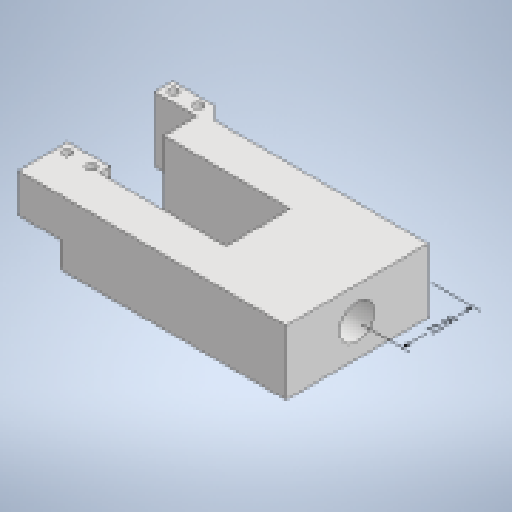
# Autodesk Inventor part: Base Catapulta
Saved by Autodesk Inventor 2024 (Build 280153000, 153)
## iProperties
Created: 2025-03-01
Part Number: Base Catapulta
Material: Genérico
Document SubType Name: Modeling
Designer: sergi
Density: 1 g/cm^3
Appearance: Valor por defecto
Author: sergi
Autodesk Inventor part; units mm, degrees
ref_plane "YZ Plane" through (0, 0, 0) normal (1, 0, 0) x (0, 1, 0)
ref_plane "XZ Plane" through (0, 0, 0) normal (0, 1, 0) x (-1, 0, 0)
ref_plane "XY Plane" through (0, 0, 0) normal (0, 0, 1) x (1, 0, 0)
sketch "Boceto1" plane through (0, 0, 0) normal (0, 1, 0) x (-1, 0, 0)
  line L0 (0, 0) -> (105, 0)
  line L1 (105, 0) -> (105, 66)
  line L2 (105, 66) -> (0, 66)
  line L3 (0, 66) -> (0, 0)
  dimension "d0" = 105
  dimension "d1" = 66
  constraints: 8 end point, 2 parallel, 1 horizontal, 1 perpendicular
  measures "d0" distance of L2.end L1.end
  measures "d1" distance of L1.end L0.end
extrude "Extrusión1" add sketch "Boceto1" along normal blind 30
sketch "Boceto2" plane through (0, 0, 66) normal (1, 0, 0) x (0, 0, -1)
  line L0 (66, 30) -> (0, 30) projected
  line L1 (0, 0) -> (66, 0) projected
  line L2 (66, 0) -> (66, 30) projected
  line L3 (0, 30) -> (66, 30) projected
  line L4 (0, 0) -> (0, 30) projected
  line L5 (66, 30) -> (0, 0)
  circle A0 centre (33, 15) radius 8.1
  dimension "d28" = 16.2
  constraints: 2 end point, 1 centre point, 1 midpoint
  measures "d28" diameter of A0
hole "Agujero1" at (0, 15, 33) direction (-1, 0, 0) diameter 16.2 depth 44
sketch "Boceto5" plane through (0, 30, 0) normal (0, 1, 0) x (1, 0, 0)
  line L0 (-105, 0) -> (-105, -66) projected
  line L1 (-105, -66) -> (0, -66) projected
  line L2 (0, -66) -> (0, 0) projected
  line L3 (0, 0) -> (-105, 0) projected
  line L4 (0, -24.9) -> (0, -41.1) projected
  line L5 (-44, -41.1) -> (-44, -24.9) projected
  line L6 (0, -41.1) -> (-44, -41.1)
  line L7 (-44, -24.9) -> (0, -24.9)
  line L8 (-46, -22.9) -> (-46, -43.1)
  line L9 (-46, -43.1) -> (2, -43.1)
  line L10 (2, -43.1) -> (2, -22.9)
  line L11 (2, -22.9) -> (-46, -22.9)
  line L12 (-46, -43.1) -> (-105, -43.1)
  line L13 (-105, 0) -> (-105, -66) projected
  line L14 (-46, -22.9) -> (-105, -22.9)
  line L15 (-105, -22.9) -> (-46, -43.1)
  line L16 (-46, -48) -> (-105, -48)
  line L17 (-105, -48) -> (-105, -18)
  line L18 (-105, -18) -> (-46, -18)
  line L19 (-46, -18) -> (-46, -48)
  line L20 (-46, -48) -> (-105, -18) construction
  line L21 (-105, -48) -> (-46, -18) construction
  point P0 (-75.5, -33)
  point P1 (-105, -18)
  dimension "d29" = 2
  dimension "d30" = 30
  constraints: 30 end point, 5 perpendicular, 4 parallel, 3 midpoint, 3 point on line, 1 horizontal, 3 other
  measures "d29" distance between parallel lines of L5 L8
  measures "d30" distance between parallel lines of L16 L18
extrude "Extrusión3" cut sketch "Boceto5" against normal through all contours L18 L19 L14 L0 | L15 L12 L0 | L14 L8 L15 | L12 L19 L16 L0
sketch "Boceto6" plane through (-46, 30, 18) normal (-1, 0, 0) x (0, 0, 1)
  circle A0 centre (20, -15) radius 1 projected
  circle A1 centre (10, -15) radius 1 projected
  point P0 (-18, -30)
hole "Agujero3" at (-46, 15, 38) at (-46, 15, 28) direction (1, 0, 0) diameter 2.2 depth 44
sketch "Boceto7" plane through (-105, 0, 66) normal (-1, 0, 0) x (0, 0, 1)
  line L0 (-18, 30) -> (-18, 0) projected
  line L1 (-18, 0) -> (0, 0) projected
  line L2 (0, 0) -> (0, 30) projected
  line L3 (-18, 30) -> (0, 30) projected
  line L4 (-68.75, 30) -> (-68.75, 32.5) projected
  line L5 (-63.6, 30) -> (-68.75, 30) projected
  line L6 (-63.6, 1.45) -> (-63.6, 30) projected
  line L7 (-23.1, 1.45) -> (-63.6, 1.45) projected
  line L8 (-23.1, 30) -> (-23.1, 1.45) projected
  line L9 (-17.95, 30) -> (-23.1, 30) projected
  line L10 (-17.95, 32.5) -> (-17.95, 30) projected
  line L11 (-23.1, 32.5) -> (-17.95, 32.5) projected
  line L12 (-23.1, 38.25) -> (-23.1, 32.5) projected
  line L13 (-33, 38.25) -> (-23.1, 38.25) projected
  line L14 (-63.6, 38.25) -> (-33, 38.25) projected
  line L15 (-63.6, 32.5) -> (-63.6, 38.25) projected
  line L16 (-68.75, 32.5) -> (-63.6, 32.5) projected
  line L17 (-23.1, 5.2) -> (-23.1, 9) projected
  line L18 (-23.1, 5.2) -> (-19.2, 5.2) projected
  line L19 (-19.2, 9) -> (-19.2, 5.2) projected
  line L20 (-23.1, 9) -> (-19.2, 9) projected
  line L21 (-23.1, 9) -> (-23.1, 12)
  line L22 (-23.1, 12) -> (0, 12)
  line L23 (-48, 0) -> (-48, 30) projected
  line L24 (-66, 30) -> (-48, 30) projected
  line L25 (-66, 0) -> (-66, 30) projected
  line L26 (-66, 0) -> (-48, 0) projected
  line L27 (-70.75, 32.5) -> (-64.75, 33.85)
  line L28 (-70.75, 32.5) -> (-70.75, 30)
  line L29 (-70.75, 32.5) -> (-70.75, 30)
  line L30 (-70.75, 30) -> (-63.6, 30)
  line L31 (-63.6, 30) -> (-63.6, 0)
  line L32 (-63.6, 0) -> (-71.95, 0)
  line L33 (-70.75, 0) -> (-70.75, 30)
  line L34 (-71.95, 31.2) -> (-62.4, 31.2)
  line L35 (-62.4, 31.2) -> (-62.4, -1.2)
  line L36 (-62.4, -1.2) -> (-71.95, -1.2)
  line L37 (-71.95, -1.2) -> (-71.95, 31.2)
  line L38 (-70.75, 0) -> (-71.95, 0)
  line L39 (-70.75, 30) -> (-71.95, 30)
  dimension "d42" = 3
  dimension "d55" = 1.2
  constraints: 30 end point, 6 point on line, 4 parallel, 4 perpendicular, 2 horizontal, 2 vertical, 5 other
  measures "d42" distance of L17.end L21.end
  measures "d55" distance between parallel lines of L33 L37
ref_plane "Plano de trabajo1" through (-124.8, 1.45, -2.75) normal (-1, 0, 0) x (0, 0, 1)
extrude "Extrusión4" add sketch "Boceto7" along normal up to surface (19.8 mm away) contours L3 L2 L22 L0 | L0 L22 L8 L9 | L31 L26 L25 L5 L6 | L25 L32 L33 L30 L5 | L32 L37 L39 L33
chamfer "Chaflán1" distance 5.95 angle 45 1 edges at (-105, 15, 0)
sketch "Boceto8" plane through (0, 30, 0) normal (0, 1, 0) x (1, 0, 0)
  circle A0 centre (-120.6, -47.5) radius 2.2 projected
  circle A1 centre (-109.2, -47.5) radius 2.2 projected
  circle A2 centre (-109.2, 2.2) radius 2.2 projected
  circle A3 centre (-120.6, 2.2) radius 2.2 projected
  point P0 (0, 0)
hole "Agujero4" at (-120.6, 30, 47.5) at (-109.2, 30, 47.5) at (-120.6, 30, -2.2) at (-109.2, 30, -2.2) direction (0, -1, 0) diameter 4.2 end through all
sketch "Boceto9" plane through (-105, 0, 66) normal (0, 0, 1) x (1, 0, 0)
  line L0 (100, 46.82) -> (91.8, 46.82) projected
  line L1 (91.8, 46.82) -> (91.8, 55.02) projected
  line L2 (91.8, 55.02) -> (100, 55.02) projected
  line L3 (100, 55.02) -> (100, 46.82) projected
  line L4 (91.8, 95) -> (100, 95) projected
  line L5 (100, 95) -> (100, 86.8) projected
  line L6 (100, 86.8) -> (91.8, 86.8) projected
  line L7 (91.8, 86.8) -> (91.8, 95) projected
  line L8 (105, 100) -> (90, 100) projected
  line L9 (90, 100) -> (70, 30) projected
  line L10 (70, 30) -> (105, 30) projected
  line L11 (105, 30) -> (105, 100) projected
  line L12 (0, 0) -> (105, 0) projected
  line L13 (105, 0) -> (105, 30) projected
  line L14 (105, 30) -> (-19.8, 30) projected
  line L15 (-19.8, 30) -> (-19.8, 12) projected
  line L16 (0, 12) -> (-19.8, 12) projected
  line L17 (0, 0) -> (0, 12) projected
  line L18 (70, 30) -> (70, 20)
  line L19 (70, 20) -> (105, 20)
  dimension "d56" = 10
  constraints: 4 end point, 2 perpendicular
  measures "d56" distance of L9.end L18.end
ref_plane "Plano de trabajo2" through (-35, 30, 56) normal (0, 0, -1) x (0, 1, 0)
extrude "Extrusión5" cut sketch "Boceto9" against normal up to surface (10 mm away) contours L13 L19 L18 L10
sketch "Boceto10" plane through (-35, 30, 56) normal (0, 0, 1) x (1, 0, 0)
  line L0 (0, -10) -> (35, -10) projected
  line L1 (35, 0) -> (-64.05, 0) projected
  line L2 (0, -10) -> (10, -10)
  line L3 (10, -10) -> (10, 0)
  line L4 (10, 0) -> (0, 0)
  line L5 (0, 0) -> (0, -10)
  line L6 (35, 0) -> (35, -10) projected
  line L7 (35, -10) -> (25, -10)
  line L8 (25, -10) -> (25, 0)
  line L9 (25, 0) -> (35, 0)
  line L10 (35, 0) -> (35, -10)
  line L11 (0, 0) -> (10, -10)
  line L12 (25, -10) -> (35, 0)
  circle A0 centre (5, -5) radius 2.1
  circle A1 centre (30, -5) radius 2.1
  point P0 (35, -30)
  dimension "d59" = 4.2
  dimension "d60" = 4.2
  constraints: 20 end point, 4 parallel, 3 perpendicular, 2 centre point, 2 horizontal, 2 midpoint, 2 point on line
  measures "d59" diameter of A0
  measures "d60" diameter of A1
hole "Agujero5" at (-30, 25, 56) at (-5, 25, 56) direction (0, 0, -1) diameter 4.2 depth 10
ref_plane "Plano de trabajo3" through (-105, 0, 33) normal (0, 0, 1) x (1, 0, 0)
mirror "Simetría1" about plane through (-105, 0, 33) normal (0, 0, 1) of "Extrusión5", "Agujero5"
